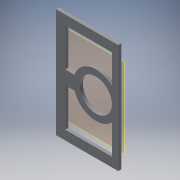
# Autodesk Inventor part: 00_PDMS_chamber_clamp
Saved by Autodesk Inventor 2019.4 (Build 234330000, 330)
## iProperties
Created: 2021-04-19
Part Number: 00_PDMS_chamber_clamp
Material: Generic
Document SubType Name: Modeling
Designer: diederichbenedict
Density: 1 g/cm^3
Appearance: Olive Green
Author: diederichbenedict
Autodesk Inventor part; units mm, degrees
ref_plane "YZ Plane" through (0, 0, 0) normal (1, 0, 0) x (0, 1, 0)
ref_plane "XZ Plane" through (0, 0, 0) normal (0, 1, 0) x (-1, 0, 0)
ref_plane "XY Plane" through (0, 0, 0) normal (0, 0, 1) x (1, 0, 0)
ref_plane "Work Plane1" through (0, 0, 0) normal (0, 0, 1) x (1, 0, 0)
sketch "Sketch1" plane through (0, 0, 0) normal (0, 0, 1) x (1, 0, 0)
  circle A0 centre (-5, 7.7) radius 2.5 projected
  circle A1 centre (-5, -7.7) radius 2.5 projected
  circle A2 centre (1.841, 0.036) radius 5 projected
  line L0 (9, 11.7) -> (-9, 11.7) construction
  line L1 (-9, 11.7) -> (-9, -11.7) construction
  line L2 (-9, -11.7) -> (9, -11.7) construction
  line L3 (9, -11.7) -> (9, 11.7) construction
  line L4 (-10.9833, 17.5) -> (-7.9833, 17.5)
  line L5 (-10.9833, -17.5) -> (-10.9833, 17.5) construction
  line L6 (-7.9833, 14.5) -> (-7.9833, 17.5) construction
  circle A3 centre (1.841, 0.036) radius 5.1595
  line L7 (7, 5.0365) -> (7, 14.5)
  line L8 (7, -14.5) -> (7, -4.9645)
  line L9 (7, -0.0344) -> (7, 0.1065)
  line L10 (-5, -2.1595) -> (-7.9833, -2.1595)
  line L11 (-5, 2.2316) -> (-7.9833, 2.2316)
  arc A4 (7, 5.0365) -> (-5, 2.2316) centre (1.841, 0.036) ccw
  arc A5 (-5, -2.1595) -> (7, -4.9645) centre (1.841, 0.036) ccw
  line L12 (-7.9833, 14.5) -> (-7.9833, 2.2316)
  line L13 (-7.9833, -2.1595) -> (-7.9833, -14.5)
  line L14 (-7.9833, -17.5) -> (-7.9833, -17.5)
  line L15 (-7.9833, 14.5) -> (7, 14.5)
  line L16 (-7.9833, -14.5) -> (7, -14.5)
  line L17 (-10.9833, 17.5) -> (9.0167, 17.5)
  line L18 (9.0167, 17.5) -> (9.0167, -17.5)
  line L19 (9.0167, -17.5) -> (-10.9833, -17.5)
  line L20 (-10.9833, -17.5) -> (-10.9833, 17.5)
  point P0 (0, 0)
  dimension "d0" = 3
  dimension "d1" = 35
  dimension "d2" = 5.8
  dimension "d7" = 20
  constraints: 34 end point, 10 perpendicular, 6 point on circle, 5 parallel, 4 horizontal, 3 centre point, 2 coincident
  measures "d0" distance of L14.end L5.start
  measures "d1" distance of L4.end L14.end
  measures "d2" distance between parallel lines of L0 L4
  measures "d7" distance of L18.end L19.end
extrude "Extrusion1" add sketch "Sketch1" along normal blind 1 contours L4 L17 L18 L19 L20
sketch "Sketch2" plane through (0, 0, 1) normal (0, 0, 1) x (1, 0, 0)
  line L0 (-7.9833, -2.1595) -> (-5, -2.1595) projected
  arc A0 (-5, -2.1595) -> (7, -4.9645) centre (1.841, 0.036) ccw projected
  line L1 (7, -4.9645) -> (7, -14.5) projected
  line L2 (7, -14.5) -> (-7.9833, -14.5) projected
  line L3 (-7.9833, -14.5) -> (-7.9833, -2.1595) projected
  arc A1 (7, 5.0365) -> (-5, 2.2316) centre (1.841, 0.036) ccw projected
  line L4 (-5, 2.2316) -> (-7.9833, 2.2316) projected
  line L5 (-7.9833, 2.2316) -> (-7.9833, 14.5) projected
  line L6 (-7.9833, 14.5) -> (7, 14.5) projected
  line L7 (7, 14.5) -> (7, 5.0365) projected
  line L8 (9.0167, 17.5) -> (-10.9833, 17.5) projected
  line L9 (-10.9833, 17.5) -> (-10.9833, -17.5) projected
  line L10 (-10.9833, -17.5) -> (9.0167, -17.5) projected
  line L11 (9.0167, -17.5) -> (9.0167, 17.5) projected
  circle A2 centre (1.841, 0.036) radius 5.1595 projected
  circle A3 centre (-13.159, 0.036) radius 1.6
  circle A4 centre (0, 20.036) radius 1.6
  circle A5 centre (0, -19.964) radius 1.6
  arc A6 (3.6, 20.036) -> (-3.6, 20.036) centre (0, 20.036) ccw
  arc A7 (-3.6, -19.964) -> (3.6, -19.964) centre (0, -19.964) ccw
  line L12 (3.6, 20.036) -> (3.6, 17.5)
  line L13 (-3.6, 20.036) -> (-3.6, 17.5)
  line L14 (-13.159, 3.636) -> (-10.9833, 3.636)
  line L15 (-13.159, -3.564) -> (-10.9833, -3.564)
  line L16 (-3.6, -19.964) -> (-3.6, -17.5)
  line L17 (3.6, -19.964) -> (3.6, -17.5)
  arc A8 (-13.159, 3.636) -> (-13.159, -3.564) centre (-13.159, 0.036) ccw
  arc A9 (-10.9833, -2.8321) -> (-10.306, -2.1595) centre (-13.159, 0.036) ccw
  arc A10 (-10.306, 2.2316) -> (-10.9833, 2.9042) centre (-13.159, 0.036) ccw
  point P0 (0, 0)
  dimension "d10" = 3.2
  dimension "d11" = 3.2
  dimension "d12" = 3.2
  dimension "d13" = 20
  dimension "d14" = 20
  dimension "d15" = 15
  dimension "d16" = 2
  dimension "d18" = 2
  constraints: 14 point on line, 12 end point, 10 point on circle, 8 centre point, 3 perpendicular, 1 parallel
  measures "d10" diameter of A3
  measures "d11" diameter of A4
  measures "d12" diameter of A5
  measures "d13" vertical distance of A4.centre A0.centre
  measures "d14" vertical distance of A0.centre A5.centre
  measures "d15" distance of A3.centre A0.centre
  measures "d16" radial gap between concentric circles of A4 A6
  measures "d18" radial gap between concentric circles of A5 A7
extrude "Extrusion2" add sketch "Sketch2" against normal blind 1 contours L8 L13 A6 L12 | L17 A7 L16 L10 | L9 L15 A8 L14
body "Solid1"
